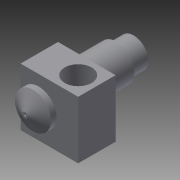
# Autodesk Inventor part: Nozzle
Saved by Autodesk Inventor 2014 SP1 (Build 180222100, 222)
## iProperties
Created: 2013-12-29
Part Number: Nozzle
Material: Brass, Soft Yellow
Document SubType Name: Modeling
Designer: Jack
Density: 8.47 g/cm^3
Appearance: Brass - Satin
Author: Jack
Autodesk Inventor part; units mm, degrees
ref_plane "YZ Plane" through (0, 0, 0) normal (1, 0, 0) x (0, 1, 0)
ref_plane "XZ Plane" through (0, 0, 0) normal (0, 1, 0) x (-1, 0, 0)
ref_plane "XY Plane" through (0, 0, 0) normal (0, 0, 1) x (1, 0, 0)
sketch "Sketch1" plane through (0, 0, 0) normal (0, 1, 0) x (-1, 0, 0)
  line L0 (0, 0) -> (12.7, 0)
  line L1 (12.7, 0) -> (12.7, 12.7)
  line L2 (12.7, 12.7) -> (0, 12.7)
  line L3 (0, 12.7) -> (0, 0)
  dimension "d0" = 12.7
  dimension "d1" = 12.7
  constraints: 8 end point, 2 perpendicular, 1 horizontal, 1 parallel
  measures "d0" distance of L0.start L0.end
  measures "d1" distance of L0.end L1.end
extrude "Extrusion1" add sketch "Sketch1" along normal blind 8.255
sketch "Sketch2" plane through (0, 8.255, 0) normal (0, 1, 0) x (1, 0, 0)
  line L0 (0, 0) -> (-12.7, 0) projected
  line L1 (-12.7, 0) -> (-12.7, -12.7) projected
  circle A0 centre (-8.7313, -6.35) radius 3.9688
  dimension "d4" = 7.9375
  dimension "d5" = 6.35
  constraints: 1 centre point, 1 tangent
  measures "d4" diameter of A0
  measures "d5" distance from line of L0 A0.centre
extrude "Extrusion2" add sketch "Sketch2" along normal blind 8.89
sketch "Sketch3" plane through (-8.7313, 17.145, 6.35) normal (0, 1, 0) x (1, 0, 0)
  circle A0 centre (0, 0) radius 3.9687 projected
  circle A1 centre (0, 0) radius 3.2385
  point P0 (8.7313, 6.35)
  dimension "d8" = 6.477
  constraints: 1 centre point, 1 coincident
  measures "d8" diameter of A1
extrude "Extrusion3" add sketch "Sketch3" along normal blind 3.81 contours A1
sketch "Sketch4" plane through (0, 0, 0) normal (0, -1, 0) x (1, 0, 0)
  circle A0 centre (-8.7313, 6.35) radius 3.9687 projected
  circle A1 centre (-8.7313, 6.35) radius 3.9688
  dimension "d11" = 7.9375
  constraints: 1 centre point, 1 coincident
  measures "d11" diameter of A1
extrude "Extrusion4" add sketch "Sketch4" along normal blind 1.27
ref_plane "Work Plane1" through (-8.7313, -3.048, 6.35) normal (0, -1, 0) x (1, 0, 0)
sketch "Sketch5" plane through (-8.7313, -3.048, 6.35) normal (0, -1, 0) x (1, 0, 0)
  circle A0 centre (0, 0) radius 3.9687 projected
  circle A1 centre (0, 0) radius 0.635
  point P0 (8.7313, -6.35)
  dimension "d16" = 1.27
  constraints: 1 centre point, 1 coincident
  measures "d16" diameter of A1
sketch "Sketch6" plane through (-8.7313, -1.27, 6.35) normal (0, -1, 0) x (1, 0, 0)
  circle A0 centre (0, 0) radius 3.9687 projected
  point P0 (8.7313, -6.35)
loft "Loft1" add profiles "Sketch5" section 1 edges at (-12.7, -1.27, 6.35) contours A1
sketch "Sketch7" plane through (-12.7, 0, 12.7) normal (0, 0, 1) x (1, 0, 0)
  line L0 (12.7, 0) -> (12.7, 8.255) projected
  line L1 (0, 8.255) -> (12.7, 8.255) projected
  circle A0 centre (8.5725, 4.1275) radius 2.9718
  dimension "d21" = 5.9436
  dimension "d22" = 4.1275
  dimension "d23" = 4.1275
  constraints: 1 centre point
  measures "d21" diameter of A0
  measures "d22" distance from line of L1 A0.centre
  measures "d23" distance from line of L0 A0.centre
extrude "Extrusion5" cut sketch "Sketch7" against normal blind 12.73
sketch "Sketch8" plane through (-12.7, 0, 12.7) normal (-1, 0, 0) x (0, 0, 1)
  line L0 (-12.7, 8.255) -> (-6.35, 8.255) projected
  line L1 (-12.7, 0) -> (-12.7, 8.255) projected
  circle A0 centre (-10.922, 4.1275) radius 1.143
  dimension "d26" = 2.286
  dimension "d27" = 4.1275
  dimension "d28" = 1.778
  constraints: 1 centre point
  measures "d26" diameter of A0
  measures "d27" distance from line of L0 A0.centre
  measures "d28" distance from line of L1 A0.centre
extrude "Extrusion6" cut sketch "Sketch8" against normal blind 4.318
sketch "Sketch9" plane through (-8.7313, 20.955, 6.35) normal (0, 1, 0) x (1, 0, 0)
  circle A0 centre (0, 0) radius 3.2385 projected
  circle A1 centre (0, 0) radius 1.7526
  point P0 (8.7313, 6.35)
  dimension "d31" = 3.5052
  constraints: 1 centre point, 1 coincident
  measures "d31" diameter of A1
extrude "Extrusion7" cut sketch "Sketch9" against normal blind 22.932 contours A1
sketch "Sketch10" plane through (-8.7313, -3.048, 6.35) normal (0, -1, 0) x (1, 0, 0)
  circle A0 centre (0, 0) radius 0.635 projected
  circle A1 centre (0, 0) radius 0.254
  point P0 (8.7313, -6.35)
  dimension "d34" = 0.508
  constraints: 1 centre point, 1 coincident
  measures "d34" diameter of A1
extrude "Extrusion8" cut sketch "Sketch10" against normal blind 6.568 contours A1
body "Solid1"
